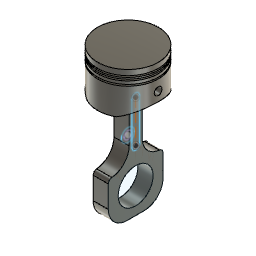
PISTON (Autodesk Fusion 360 design; units mm, degrees)
Autodesk Fusion 360 part; units mm, degrees
sketch "Sketch1" plane through (0, 0, 0) normal (0, 1, 0) x (1, 0, 0) in component "piston"
  line L0 (0, 0) -> (0, -55)
  line L1 (0, -55) -> (-40, -55)
  line L2 (-40, -55) -> (-40, -48)
  line L3 (-40, -48) -> (-36, -48)
  line L4 (-36, -48) -> (-36, -46)
  line L5 (-36, -46) -> (-40, -46)
  line L6 (-40, -46) -> (-40, -44)
  line L7 (-40, -44) -> (-36, -44)
  line L8 (-36, -44) -> (-36, -42)
  line L9 (-36, -42) -> (-40, -42)
  line L10 (-40, -42) -> (-40, -38)
  line L11 (-40, -38) -> (-36, -38)
  line L12 (-36, -38) -> (-36, -36)
  line L13 (-36, -36) -> (-40, -36)
  line L14 (-40, -36) -> (-40, 0)
  line L15 (0, 0) -> (-40, 0)
  dimension "d1" = 40
  dimension "d2" = 7
  dimension "d3" = 4
  dimension "d4" = 2
  dimension "d5" = 2
  dimension "d6" = 4
  dimension "d7" = 2
  dimension "d8" = 4
  dimension "d9" = 2
  dimension "d10" = 36
  dimension "d11" = 4
  constraint coincident L0.start L15.start
  constraint vertical L0
  constraint perpendicular L0 L1
  constraint perpendicular L1 L2
  constraint perpendicular L2 L3
  constraint perpendicular L1 L4
  constraint perpendicular L4 L5
  constraint perpendicular L1 L6
  constraint perpendicular L6 L7
  constraint perpendicular L7 L8
  constraint perpendicular L8 L9
  constraint perpendicular L9 L10
  constraint perpendicular L10 L11
  constraint perpendicular L11 L12
  constraint perpendicular L10 L13
  constraint perpendicular L11 L14
  constraint perpendicular L14 L15
  measures "d1" distance of L0.end L1.end
  measures "d2" distance of L1.end L2.end
  measures "d3" distance of L2.end L3.end
  measures "d4" distance of L3.end L4.end
  measures "d5" distance of L5.end L6.end
  measures "d6" distance of L6.end L7.end
  measures "d7" distance of L7.end L8.end
  measures "d8" distance of L9.end L10.end
  measures "d9" distance of L11.end L12.end
  measures "d10" distance of L13.end L14.end
  measures "d11" distance of L10.end L11.end
revolve "Revolve1" add sketch "Sketch1" angle 360 about axis through (0, 0, 0) along (0, 0, 1) makes body 1 in component "piston"
sketch "Sketch2" plane through (0, 0, 0) normal (1, 0, 0) x (0, 1, 0) in component "piston"
  line L0 (0, 1.75) -> (0, 22.5)
  arc A0 (35, 0) -> (-35, 0) centre (0, -56.25) ccw
  line L1 (35, 0) -> (-35, 0)
  point P0 (0, 10)
  point P1 (-35, 0)
  point P2 (-39.5, 0)
  point P3 (35, 0)
  point P4 (39.5, 0)
  dimension "d13" = 10
  dimension "d14" = 4.5
  constraint horizontal P1 P2
  constraint symmetric P1 L0 P3
  constraint symmetric P2 L0 P4
  constraint coincident P0 A0
  constraint coincident P1 A0.end
  constraint coincident P3 A0.start
  measures "d13" distance of origin P0
  measures "d14" distance of P1 P2
sketch "Sketch3" plane through (0, 0, 0) normal (0, 0, -1) x (1, 0, 0) in component "piston"
  circle A0 centre (0, 0) radius 40
  circle A1 centre (0, 0) radius 32.6956
  constraint concentric A0 A1
extrude "Extrude2" cut sketch "Sketch3" against normal blind 36 contours A1 bodies 1 in component "piston"
extrude "Extrude1" cut sketch "Sketch2" along normal mid plane 106 bodies 1 in component "piston"
sketch "Sketch4" plane through (0, 0, 0) normal (1, 0, 0) x (0, 1, 0) in component "piston"
  circle A0 centre (0, 22) radius 5
extrude "Extrude3" cut sketch "Sketch4" along normal mid plane 200 bodies 1 in component "piston"
sketch "Sketch5" plane through (0, 0, 0) normal (1, 0, 0) x (0, 1, 0) in component "piston"
sketch "Sketch6" plane through (0, 0, 0) normal (1, 0, 0) x (0, 1, 0) in component "piston"
sketch "Sketch1 (2)" plane through (0, 0, 0) normal (1, 0, 0) x (0, 1, 0) in component "connecting rod"
  spline S0 degree 3 poles (-5, 22) (-5, 22.6285) (-4.8743, 23.2985) (-4.3638, 24.5302) (-3.9791, 25.092) (-3.092, 25.9791) (-2.5302, 26.3638) (-1.2985, 26.8743) (-0.6285, 27) (0.6285, 27) (1.2985, 26.8743) (2.5302, 26.3638) (3.092, 25.9791) (3.9791, 25.092) (4.3638, 24.5302) (4.8743, 23.2985) (5, 22.6285) (5, 21.3715) (4.8743, 20.7015) (4.3638, 19.4698) (3.9791, 18.908) (3.092, 18.0209) (2.5302, 17.6362) (1.2985, 17.1257) (0.6285, 17) (-0.6285, 17) (-1.2985, 17.1257) (-2.5302, 17.6362) (-3.092, 18.0209) (-3.9791, 18.908) (-4.3638, 19.4698) (-4.8743, 20.7015) (-5, 21.3715) (-5, 22) knots 0 0 0 0 0.188556 0.188556 0.377112 0.377112 0.565667 0.565667 0.754221 0.754221 0.942775 0.942775 1.13133 1.13133 1.319886 1.319886 1.508442 1.508442 1.696998 1.696998 1.885554 1.885554 2.074108 2.074108 2.262663 2.262663 2.451217 2.451217 2.639772 2.639772 2.828328 2.828328 3.016884 3.016884 3.016884 3.016884
  circle A0 centre (0, 22) radius 8.5
  dimension "d21" = 17
  measures "d21" diameter of A0
sketch "Sketch2 (2)" plane through (0, 0, 0) normal (1, 0, 0) x (0, 1, 0) in component "connecting rod"
  line L0 (0, 22) -> (0, -101)
  circle A0 centre (0, -101) radius 23
  line L1 (36, -76) -> (36, -101)
  line L2 (0, -101) -> (36, -101)
  circle A1 centre (0, 22) radius 8.5
  line L3 (8.5, 22.0114) -> (8.598, -51.0165)
  line L4 (33.4266, -75.9823) -> (36, -76)
  line L5 (8.6313, -75.8123) -> (8.6306, -75.2712)
  arc A2 (8.598, -51.0165) -> (33.4266, -75.9823) centre (33.598, -50.9829) ccw
  line L6 (-8.5, 22.0114) -> (-8.598, -51.0165)
  arc A3 (-33.4266, -75.9823) -> (-8.598, -51.0165) centre (-33.598, -50.9829) ccw
  line L7 (-36, -76) -> (-36, -101)
  line L8 (0, -101) -> (-36, -101)
  line L9 (-33.4266, -75.9823) -> (-36, -76)
  line L10 (-36, -101) -> (-36, -135)
  line L11 (-36, -135) -> (36.3575, -135)
  line L12 (36.3575, -135) -> (36, -101)
  point P0 (0, 22)
  dimension "d22" = 123
  dimension "d23" = 46
  dimension "d24" = 36
  dimension "d25" = 25
  dimension "d26" = 25
  constraint coincident P0 L0.start
  constraint vertical L0
  constraint coincident L0.end A0.centre
  constraint vertical L1
  constraint perpendicular L1 L2
  constraint coincident A1 L3.start
  constraint tangent A1 L3
  constraint coincident L3 L5.end
  constraint coincident L5.start L3
  constraint coincident L5.start L4
  constraint tangent L3 A2
  constraint tangent L4 A2
  constraint symmetric L0 L1.start L7.start
  constraint symmetric L0 A0.centre L2.start
  constraint symmetric L0 L1.end L7.end
  constraint symmetric L0 L3.start L6.start
  constraint symmetric L0 L3.end L6.end
  constraint symmetric L0 L4.start A3.start
  constraint symmetric L0 A2 A3
  constraint perpendicular L8 L10
  constraint perpendicular L7 L11
  measures "d22" distance of P0 L0.end
  measures "d23" diameter of A0
  measures "d24" distance of L0 L1
  measures "d25" distance of L1.start L1.end
  measures "d26" radius of A2
extrude "Extrude1'" add sketch "Sketch2 (2)" along normal mid plane 20 separate body contours L0 A0 L1 L2 A1 L3 L4 A2 | L0 A0 A1 L6 A3 L7 L8 L9 | A0 L2 L8 L10 L11 L12 makes body 2 in component "connecting rod"
fillet "Fillet1" radius 25 2 edges at (0, -36, -135) (0, 36.3575, -135) on bodies 2 in component "connecting rod"
fillet "Fillet2" radius 5 2 edges at (0, 36, -76) (0, -36, -76) on bodies 2 in component "connecting rod"
move_body "Move1" bodies 1 to x (1, 0, 0) y (0, 1, 0) z (0, 0, 1) at (0, 0, 70) in component "piston"
move_body "Move1'" bodies 2 to x (1, 0, 0) y (0, 1, 0) z (0, 0, 1) at (0, 0.094, 69.9999) in component "connecting rod"
sketch "Sketch7" plane through (10, 0, 0) normal (1, 0, 0) x (0, 1, 0) in component "piston"
  arc A0 (-31.339, -5.8891) -> (-35.906, -10.8703) centre (-30.906, -10.8703) ccw
  line L0 (-35.906, -10.8703) -> (-35.906, -40.0001)
  arc A1 (-35.906, -40.0001) -> (-10.906, -65.0001) centre (-10.906, -40.0001) ccw
  line L1 (-10.906, -65.0001) -> (11.1872, -65.0001)
  arc A2 (11.1872, -65.0001) -> (36.1859, -39.7372) centre (11.1872, -40.0001) ccw
  line L2 (36.1859, -39.7372) -> (36.094, -31.0001)
  line L3 (36.094, -31.0001) -> (36.094, -10.8703)
  arc A3 (36.094, -10.8703) -> (31.527, -5.8891) centre (31.094, -10.8703) ccw
  arc A4 (8.692, 18.9834) -> (31.527, -5.8891) centre (33.692, 19.017) ccw
  line L4 (8.692, 18.9834) -> (8.594, 92.0113)
  arc A5 (-8.406, 92.0113) -> (8.594, 92.0113) centre (0.094, 91.9999) ccw
  line L5 (-8.406, 92.0113) -> (-8.5041, 18.9834)
  arc A6 (-31.339, -5.8891) -> (-8.5041, 18.9834) centre (-33.504, 19.017) ccw
  circle A7 centre (0.094, -31.0001) radius 23
  line L6 (-5, 70) -> (-5, 15)
  arc A8 (-5, 15) -> (5, 15) centre (0, 15) ccw
  line L7 (5, 15) -> (5, 70)
  arc A9 (5, 70) -> (-5, 70) centre (0, 70) ccw
  line L8 (0, 70) -> (0, 15) construction
  constraint tangent L6 A8
  constraint tangent A8 L7
  constraint parallel L6 L7
  constraint tangent L7 A9
  constraint tangent L6 A9
  constraint vertical L8
component "piston" placed x (1, 0, 0) y (0, 1, 0) z (0, 0, 1) at (0, 0, 0)
component "connecting rod" placed x (1, 0, 0) y (0, 1, 0) z (0, 0, 1) at (0, 0, 0) in component "piston"
